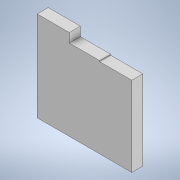
# Autodesk Inventor part: unwrappedChimney
Saved by Autodesk Inventor 2020.1 (Build 241239000, 239)
## iProperties
Created: 2019-08-11
Part Number: unwrappedChimney
Material: Generic
Document SubType Name: Modeling
Designer: steele
Density: 1 g/cm^3
Appearance: Default
Mass: 1.84433e+06 g
Surface Area: 152142 cm^2
Volume: 1.84433e+06 cm^3
Author: steele
Autodesk Inventor part; units mm, degrees
ref_plane "YZ Plane" through (0, 0, 0) normal (1, 0, 0) x (0, 1, 0)
ref_plane "XZ Plane" through (0, 0, 0) normal (0, 1, 0) x (-1, 0, 0)
ref_plane "XY Plane" through (0, 0, 0) normal (0, 0, 1) x (1, 0, 0)
sketch "Sketch1" plane through (0, 0, 0) normal (0, 0, 1) x (1, 0, 0)
  line L0 (0, 0) -> (889, 0)
  line L1 (889, 0) -> (889, 2489.2)
  line L2 (889, 2489.2) -> (0, 2489.2)
  line L3 (0, 2489.2) -> (0, 0)
  line L4 (889, 0) -> (1727.2, 0)
  line L5 (1727.2, 0) -> (1727.2, 2235.2)
  line L6 (1727.2, 2235.2) -> (889, 2235.2)
  line L7 (889, 2235.2) -> (889, 0)
  line L8 (1727.2, 0) -> (2616.2, 0)
  line L9 (2616.2, 0) -> (2616.2, 2209.8)
  line L10 (2616.2, 2209.8) -> (1727.2, 2209.8)
  line L11 (1727.2, 2209.8) -> (1727.2, 0)
  line L12 (2616.2, 0) -> (3454.4, 0)
  line L13 (3454.4, 0) -> (3454.4, 2489.2)
  line L14 (3454.4, 2489.2) -> (2616.2, 2489.2)
  line L15 (2616.2, 2489.2) -> (2616.2, 0)
  point P0 (2616.2, 1219.2)
  point P1 (1727.2, 1320.8)
  point P2 (889, 1219.2)
  dimension "d0" = 889
  dimension "d1" = 2489.2
  dimension "d2" = 838.2
  dimension "d3" = 2235.2
  dimension "d4" = 889
  dimension "d5" = 2209.8
  dimension "d6" = 838.2
  dimension "d7" = 2489.2
  dimension "d10" = 3454.4
  constraints: 32 end point, 8 parallel, 4 horizontal, 4 perpendicular
  measures "d0" distance of L2.end L1.end
  measures "d1" distance of L1.end L0.end
  measures "d2" distance of L6.end L5.end
  measures "d3" distance of L5.end L4.end
  measures "d4" distance of L10.end L9.end
  measures "d5" distance of L9.end L8.end
  measures "d6" distance of L14.end L13.end
  measures "d7" distance of L13.end L12.end
  measures "d10" distance of L12.end L0.start
extrude "Extrusion1" add sketch "Sketch1" against normal blind 304.8 contours L3 L2 L1 L0 | L1 L6 L5 L4 | L5 L10 L9 L8
body "Solid1"
